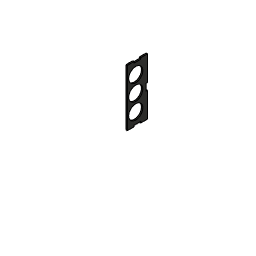
005_nixie_mounting_plate (Autodesk Fusion 360 design; units mm, degrees)
Autodesk Fusion 360 part; units mm, degrees
note: some values were not read from the file. Set by a fixed rule: which sketch regions a step uses.
sketch "Sketch1" plane through (150, 105, -5.5) normal (1, 0, 0) x (0, 0, -1)
  line L0 (-5.5, 35) -> (-7.5, 35) construction
  line L1 (-7.5, -105) -> (-5.5, -105) construction
  line L2 (8.5, 9.5) -> (-6.5, 9.5)
  line L3 (-6.5, 9.5) -> (-6.5, -32.5)
  circle A0 centre (-0.25, -11.5) radius 5.25
  circle A1 centre (-0.25, -23.5) radius 5.25
  circle A2 centre (-0.25, 0.5) radius 5.25
  line L4 (-5.5, -27.5) -> (-5.5, 12.5) construction
  line L5 (-7.5, 12.5) -> (-7.5, -27.5) construction
  line L6 (-5.5, 8.5) -> (-5.5, -23.5) construction
  line L7 (-1.5, 9.5) -> (3.5, 9.5)
  line L8 (3.5, 9.5) -> (3.5, 8.5)
  line L9 (3.5, 8.5) -> (-1.5, 8.5)
  line L10 (-1.5, 8.5) -> (-1.5, 9.5)
  line L11 (8.5, -9) -> (7.5, -9)
  line L12 (7.5, -9) -> (7.5, -14)
  line L13 (7.5, -14) -> (8.5, -14)
  line L14 (8.5, -14) -> (8.5, -9)
  line L15 (3.5, -32.5) -> (-1.5, -32.5)
  line L16 (-1.5, -32.5) -> (-1.5, -31.5)
  line L17 (-1.5, -31.5) -> (3.5, -31.5)
  line L18 (3.5, -31.5) -> (3.5, -32.5)
  line L19 (-5.5, -31.5) -> (-5.5, 8.5)
  line L20 (-5.5, 8.5) -> (-7.5, 8.5)
  line L21 (-7.5, 8.5) -> (-7.5, -31.5)
  line L22 (-7.5, -31.5) -> (-5.5, -31.5)
  line L23 (1, 8.5) -> (1, 9.5) construction
  line L24 (8.5, 9.5) -> (8.5, -32.5)
  line L25 (8.5, -32.5) -> (-6.5, -32.5)
  line L26 (1, -32.5) -> (1, -31.5) construction
  line L27 (8.5, -11.5) -> (-6.5, -11.5) construction
  dimension "d426" = 10.5
  dimension "d430" = 0
  dimension "d431" = 12
  dimension "d436" = 15
  dimension "d448" = 5
  dimension "d449" = 1
  dimension "d450" = 1
  dimension "d451" = 5
  dimension "d453" = 5
  dimension "d703" = 1
  dimension "d993" = 1
  constraint horizontal L2
  constraint vertical L3
  constraint tangent A2 L6
  constraint horizontal L7
  constraint vertical L8
  constraint horizontal L9
  constraint vertical L10
  constraint coincident L2 L7.start
  constraint horizontal L11
  constraint vertical L12
  constraint horizontal L13
  constraint vertical L14
  constraint horizontal L15
  constraint vertical L16
  constraint horizontal L17
  constraint vertical L18
  constraint collinear L9 L20
  constraint collinear L17 L22
  constraint midpoint L9 L23.start
  constraint midpoint L2 L23.end
  constraint vertical L23
  constraint perpendicular L2 L24
  constraint perpendicular L3 L25
  constraint coincident L3.end L25.end
  constraint collinear L15 L25
  constraint midpoint L25 L26.start
  constraint midpoint L17 L26.end
  constraint vertical L26
  constraint midpoint L24 L27.start
  constraint midpoint L3 L27.end
  constraint collinear L14 L24
  constraint symmetric L11 L13 L27
  constraint coincident A0.centre L27
  measures "d426" diameter of A0
  measures "d436" distance of L2.start L2.end
  measures "d448" distance of L8.end L9.end
  measures "d449" distance of L7.end L8.end
  measures "d450" distance of L11.start L11.end
  measures "d451" distance of L11.end L12.end
  measures "d453" distance of L16.end L17.end
  measures "d703" distance of L3 L4
  measures "d993" distance of L15.end L16.end
extrude "Extrude1" add sketch "Sketch1" against normal blind 1 contours L2 L3 L8 L9 L10 L11 L12 L13 L16 L17 L18 L19 L20 L22 L24 L25 | L3 L19 L20 L22
equation "d450 = d449"
equation "d451 = d448"
equation "d453 = d448"
equation "d993 = d449"
